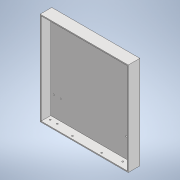
# Autodesk Inventor part: Component12
Saved by Autodesk Inventor 2022 (Build 260153000, 153)
## iProperties
Created: 2022-04-23
Part Number: Component12
Material: Generic
Document SubType Name: Modeling
Designer: Administrator
Density: 1 g/cm^3
Appearance: Default
Mass: 122.438 g
Surface Area: 645.504 cm^2
Volume: 122.438 cm^3
Title: Component12
Author: Administrator
Autodesk Inventor part; units mm, degrees
ref_plane "YZ Plane" through (0, 0, 0) normal (1, 0, 0) x (0, 1, 0)
ref_plane "XZ Plane" through (0, 0, 0) normal (0, 1, 0) x (-1, 0, 0)
ref_plane "Work Plane1" through (0, 0, 15) normal (0, 0, 1) x (1, 0, 0)
sketch "Sketch1" plane through (0, 0, 15) normal (0, 0, 1) x (1, 0, 0)
  line L0 (0, 0) -> (175, 0)
  line L1 (175, 0) -> (175, 185)
  line L2 (175, 185) -> (0, 185)
  line L3 (0, 185) -> (0, 0)
  dimension "d7" = 175
  dimension "d8" = 185
  constraints: 8 end point, 2 parallel, 1 coincident, 1 horizontal, 1 perpendicular
  measures "d7" distance of L2.end L1.end
  measures "d8" distance of L0.end L1.end
extrude "Extrusion1" add sketch "Sketch1" along normal blind 4
sketch "Sketch2" plane through (0, 0, 19) normal (0, 0, 1) x (1, 0, 0)
  line L0 (175, 185) -> (0, 185) projected
  line L1 (175, 0) -> (175, 185) projected
  line L2 (0, 185) -> (0, 0) projected
  point P0 (15.5, 179)
  point P1 (9.5, 167)
  point P2 (21.5, 167)
  point P3 (159.5, 179)
  point P4 (153.5, 167)
  point P5 (165.5, 167)
  dimension "d9" = 12
  dimension "d10" = 6
  dimension "d11" = 6
  dimension "d12" = 12
  dimension "d13" = 6
  dimension "d14" = 12
  dimension "d15" = 6
  dimension "d16" = 12
  dimension "d17" = 6
  dimension "d18" = 6
  dimension "d19" = 144
  dimension "d20" = 9.5
  dimension "d21" = 9.5
  measures "d9" vertical distance of point (9.5, 167) point (15.5, 179)
  measures "d10" horizontal distance of point (15.5, 179) point (9.5, 167)
  measures "d11" horizontal distance of point (21.5, 167) point (15.5, 179)
  measures "d12" vertical distance of point (21.5, 167) point (15.5, 179)
  measures "d13" distance from line of L0 point (15.5, 179)
  measures "d14" vertical distance of point (165.5, 167) point (159.5, 179)
  measures "d15" horizontal distance of point (159.5, 179) point (165.5, 167)
  measures "d16" vertical distance of point (153.5, 167) point (159.5, 179)
  measures "d17" horizontal distance of point (159.5, 179) point (153.5, 167)
  measures "d18" distance from line of L0 point (159.5, 179)
  measures "d19" distance of point (15.5, 179) point (159.5, 179)
  measures "d20" distance from line of L1 point (165.5, 167)
  measures "d21" distance from line of L2 point (9.5, 167)
hole "Hole1" at (15.5, 179, 19) at (9.5, 167, 19) at (21.5, 167, 19) at (159.5, 179, 19) at (153.5, 167, 19) at (165.5, 167, 19) direction (0, 0, -1) diameter 3.4 end through all clearance for "Socket Head Cap Screw" size "M3" standard "Ansi Metric M Profile"
sketch "Sketch3" plane through (0, 0, 19) normal (0, 0, 1) x (1, 0, 0)
  circle A0 centre (153.5, 167) radius 1.7 projected
  circle A1 centre (21.5, 167) radius 1.7 projected
  circle A2 centre (15.5, 179) radius 1.7 projected
  circle A3 centre (9.5, 167) radius 1.7 projected
  circle A4 centre (159.5, 179) radius 1.7 projected
  circle A5 centre (165.5, 167) radius 1.7 projected
  line L0 (175, 0) -> (175, 185) projected
  line L1 (175, 185) -> (0, 185) projected
  line L2 (0, 185) -> (0, 0) projected
  line L3 (0, 0) -> (175, 0) projected
  line L4 (2, 183) -> (173, 183)
  line L5 (173, 183) -> (173, 2)
  line L6 (173, 2) -> (2, 2)
  line L7 (2, 2) -> (2, 183)
  dimension "d34" = 2
  constraints: 8 end point, 3 other
  measures "d34" distance between parallel lines of L1 L4
extrude "Extrusion2" add sketch "Sketch3" along normal blind 19.05 contours L3 L2 L1 L0
sketch "Sketch5" plane through (0, 0, 15) normal (0, 0, -1) x (-1, 0, 0)
  line L0 (0, 0) -> (-175, 0) projected
  line L1 (0, 185) -> (0, 0) projected
  point P0 (-8.5, 41)
  point P1 (-22.5, 41)
  dimension "d38" = 14
  dimension "d39" = 8.5
  dimension "d40" = 41
  constraints: 1 horizontal alignment
  measures "d38" distance of point (-22.5, 41) point (-8.5, 41)
  measures "d39" distance from line of point (-8.5, 41) L1
  measures "d40" distance from line of L0 point (-8.5, 41)
sketch "Sketch6" plane through (0, 0, 15) normal (0, -1, 0) x (1, 0, 0)
  line L0 (0, 0) -> (0, 23.05) projected
  point P0 (0, -15)
  point P1 (8.5, 11.525)
  point P2 (22.5, 11.525)
  point P3 (0, 11.525)
  dimension "d41" = 8.5
  dimension "d42" = 14
  constraints: 2 horizontal alignment, 1 midpoint
  measures "d41" distance from line of L0 point (8.5, 11.525)
  measures "d42" distance of point (22.5, 11.525) point (8.5, 11.525)
hole "Hole2" at (8.5, 41, 15) at (22.5, 41, 15) direction (0, 0, 1) diameter 3 end through all
hole "Hole3" at (8.5, 0, 26.525) at (22.5, 0, 26.525) direction (0, 1, 0) diameter 3 depth 2
ref_plane "Work Plane2" through (87.5, 0, 15) normal (-1, 0, 0) x (0, 0, 1)
mirror "Mirror1" about plane through (87.5, 0, 15) normal (-1, 0, 0) of "Hole2", "Hole3"
sketch "Sketch7" plane through (0, 0, 15) normal (0, -1, 0) x (1, 0, 0)
  line L0 (58.5, 17.5) -> (116.5, 17.5) construction
  line L1 (0, 23.05) -> (175, 23.05) construction
  point P0 (0, -15)
  point P1 (87.5, 17.5)
  point P2 (87.5, 23.05)
  dimension "d57" = 58
  dimension "d58" = 5.55
  constraints: 2 end point, 2 midpoint, 1 horizontal, 1 vertical alignment
  measures "d57" distance of L0.start L0.end
  measures "d58" distance between parallel lines of L1 L0
hole "Hole4" at (58.5, 0, 32.5) at (116.5, 0, 32.5) direction (0, 1, 0) diameter 3 depth 2
sketch "Sketch8" plane through (0, 0, 15) normal (0, 0, -1) x (-1, 0, 0)
  line L0 (0, 0) -> (-175, 0) projected
  line L1 (-58.5, 10) -> (-116.5, 10) construction
  point P0 (-58.5, 30)
  point P1 (-116.5, 30)
  point P2 (-87.5, 10)
  point P3 (-87.5, 0)
  dimension "d66" = 58
  dimension "d67" = 10
  dimension "d68" = 20
  constraints: 3 vertical alignment, 2 end point, 2 midpoint, 1 horizontal, 1 horizontal alignment
  measures "d66" distance of L1.end L1.start
  measures "d67" distance from line of L0 L1.start
  measures "d68" distance of point (-58.5, 30) L1.start
hole "Hole5" at (58.5, 10, 15) at (58.5, 30, 15) at (116.5, 10, 15) at (116.5, 30, 15) direction (0, 0, 1) diameter 3 depth 8
equation "\"d20\" = d21"
body "Solid3"
